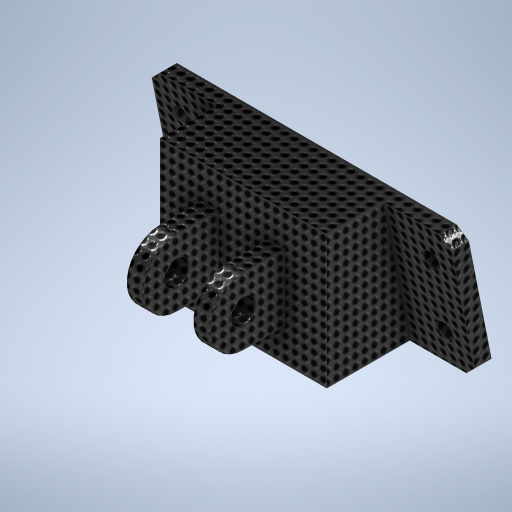
# Autodesk Inventor part: Base
Saved by Autodesk Inventor 2024 (Build 280153000, 153)
## iProperties
Created: 2023-06-06
Part Number: Base
Material: Generic
Document SubType Name: Modeling
Designer: Samyak Gosalia
Density: 1 g/cm^3
Appearance: Default
Author: Samyak Gosalia
Autodesk Inventor part; units mm, degrees
ref_plane "XZ Plane" through (0, 0, 0) normal (0, 1, 0) x (-1, 0, 0)
ref_plane "XY Plane" through (0, 0, 0) normal (0, 0, 1) x (1, 0, 0)
ref_plane "Work Plane1" through (25, 0, 0) normal (1, 0, 0) x (0, 1, 0)
sketch "Sketch1" plane through (0, 0, 0) normal (0, 0, 1) x (1, 0, 0)
  line L0 (0, 0) -> (50, 0)
  line L1 (50, 0) -> (50, 40)
  line L2 (50, 40) -> (0, 40)
  line L3 (0, 40) -> (0, 0)
  dimension "d0" = 50
  dimension "d1" = 40
  constraints: 8 end point, 2 parallel, 1 horizontal, 1 perpendicular
  measures "d0" distance of L2.end L1.end
  measures "d1" distance of L1.end L0.end
extrude "Extrusion1" add sketch "Sketch1" along normal blind 30
sketch "Sketch3" plane through (50, 0, 0) normal (1, 0, 0) x (0, 0, -1)
  line L0 (0, 0) -> (-8, 40)
  line L1 (0, 40) -> (-30, 40) projected
  line L2 (0, 0) -> (40.7922, 0) construction
  arc A0 (0, 40) -> (-8, 40) centre (-4, 20) ccw
  line L3 (0, 0) -> (0, 40) projected
  line L4 (0, 40) -> (0, 0)
  dimension "d7" = 101.31
  constraints: 6 end point, 2 point on circle, 1 centre point, 1 collinear, 1 equal length, 1 horizontal, 1 midpoint, 1 point on line
  measures "d7" angle of L2 L0
extrude "Extrusion3" cut sketch "Sketch3" against normal through all contours L0 L1 L3
sketch "Sketch4" plane through (0, 0, 30) normal (0, 0, 1) x (1, 0, 0)
  line L0 (0, 0) -> (50, 0) construction
  line L1 (25, 0) -> (25, 40) construction
  line L2 (50, 40) -> (0, 40) construction
  line L3 (0, 40) -> (0, 0) construction
  line L4 (0, 20) -> (50, 20) construction
  line L5 (50, 0) -> (50, 40) construction
  line L6 (17.5, 10) -> (17.5, 30)
  line L7 (32.5, 10) -> (32.5, 30)
  line L8 (12.5, 10) -> (12.5, 30)
  line L9 (37.5, 10) -> (37.5, 30)
  line L10 (12.5, 10) -> (17.5, 10)
  line L11 (32.5, 10) -> (37.5, 10)
  line L12 (12.5, 30) -> (17.5, 30)
  line L13 (32.5, 30) -> (37.5, 30)
  dimension "d12" = 7.5
  dimension "d13" = 7.5
  dimension "d14" = 5
  dimension "d15" = 20
  dimension "d16" = 5
  dimension "d17" = 20
  dimension "d18" = 10
  dimension "d19" = 10
  constraints: 20 end point, 7 perpendicular, 4 midpoint, 1 parallel
  measures "d12" distance between parallel lines of L6 L1
  measures "d13" distance between parallel lines of L1 L7
  measures "d14" distance of L7.end L9.end
  measures "d15" distance of L9.start L9.end
  measures "d16" distance of L8.end L6.end
  measures "d17" distance of L8.start L8.end
  measures "d18" distance between parallel lines of L0 L10
  measures "d19" distance between parallel lines of L0 L11
extrude "Extrusion4" add sketch "Sketch4" along normal blind 22.5
fillet "Fillet1" radius 10 4 edges at (15, 10, 52.5) (15, 30, 52.5) (35, 10, 52.5) (35, 30, 52.5)
sketch "Sketch5" plane through (37.5, 10, 30) normal (1, 0, 0) x (0, 0, -1)
  arc A0 (-12.5, 20) -> (-12.5, 0) centre (-12.5, 10) ccw projected
  line L0 (-12.5, 0) -> (-12.5, 20) construction
  circle A1 centre (-12.5, 10) radius 3.75
  point P0 (30, -10)
  dimension "d23" = 7.5
  constraints: 2 end point, 1 centre point, 1 coincident, 1 vertical
  measures "d23" diameter of A1
extrude "Extrusion5" cut sketch "Sketch5" against normal through all
sketch "Sketch6" plane through (25, 0, 0) normal (1, 0, 0) x (0, 1, 0)
  line L0 (40, 8) -> (40, 30) projected
  line L1 (0, 0) -> (40, 8)
  line L2 (40, 8) -> (40, 13.0991)
  line L3 (40, 13.0991) -> (0, 5.099)
  line L4 (0, 5.099) -> (0, 0)
  dimension "d27" = 5
  constraints: 8 end point, 2 parallel, 1 point on line
  measures "d27" distance between parallel lines of L1 L3
extrude "Extrusion6" add sketch "Sketch6" along normal mid plane 90
sketch "Sketch7" plane through (50, 0, 5.099) normal (0, -0.1961173, 0.9805804) x (1, 0, 0)
  circle A0 centre (12.5, 10) radius 2.5
  circle A1 centre (12.5, 30.7922) radius 2.5
  line L0 (20, 40.7922) -> (20, 0) projected
  line L1 (0, 0) -> (20, 0) projected
  line L2 (0, 40.7922) -> (20, 40.7922) projected
  point P0 (-50, -1)
  dimension "d30" = 5
  dimension "d31" = 5
  dimension "d32" = 7.5
  dimension "d33" = 7.5
  dimension "d34" = 10
  dimension "d35" = 10
  constraints: 2 centre point
  measures "d30" diameter of A0
  measures "d31" diameter of A1
  measures "d32" distance from line of L0 A0.centre
  measures "d33" distance from line of L0 A1.centre
  measures "d34" distance from line of L1 A0.centre
  measures "d35" distance from line of L2 A1.centre
extrude "Extrusion7" cut sketch "Sketch7" against normal through all
mirror "Mirror1" about plane through (25, 0, 0) normal (1, 0, 0) of "Extrusion7"
chamfer "Chamfer1" distance 3 angle 45 4 edges at (70, 0, 2.5495) (70, 40, 10.5496) (-20, 0, 2.5495) (-20, 40, 10.5496)
body "Solid1"
